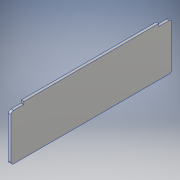
# Autodesk Inventor part: sides
Saved by Autodesk Inventor 2018.1 (Build 221171000, 171)
## iProperties
Created: 2019-02-20
Part Number: sides
Material: Aluminum 6061
Document SubType Name: Sheet Metal
Designer: RCCol
Density: 2.7 g/cm^3
Sheet Metal Rule: 3mm thick aluminum
Appearance: Aluminum - Flat
Author: RCCol
Autodesk Inventor part; units mm, degrees
ref_plane "YZ Plane" through (0, 0, 0) normal (1, 0, 0) x (0, 1, 0)
ref_plane "XZ Plane" through (0, 0, 0) normal (0, 1, 0) x (-1, 0, 0)
ref_plane "XY Plane" through (0, 0, 0) normal (0, 0, 1) x (1, 0, 0)
sketch "Sketch1" plane through (0, 0, 0) normal (1, 0, 0) x (0, 1, 0)
  line L0 (63.5, -12.7) -> (60.325, -12.7)
  line L1 (60.325, -12.7) -> (60.325, 0)
  arc A0 (60.325, 0) -> (57.15, 3.175) centre (57.15, 0) ccw
  line L2 (57.15, 3.175) -> (6.35, 3.175)
  arc A1 (6.35, 3.175) -> (3.175, 0) centre (6.35, 0) ccw
  line L3 (3.175, 0) -> (3.175, -191.77)
  arc A2 (3.175, -191.77) -> (6.35, -194.945) centre (6.35, -191.77) ccw
  line L4 (6.35, -194.945) -> (57.15, -194.945)
  arc A3 (57.15, -194.945) -> (60.325, -191.77) centre (57.15, -191.77) ccw
  line L5 (60.325, -191.77) -> (60.325, -179.07)
  line L6 (60.325, -179.07) -> (63.5, -179.07)
  line L7 (63.5, -179.07) -> (63.5, -12.7)
  line L8 (60.325, -179.07) -> (63.5, -179.07)
  line L9 (60.325, -179.07) -> (60.325, -191.77)
  line L10 (63.5, -12.7) -> (60.325, -12.7)
  line L11 (60.325, -12.7) -> (60.325, 0)
  line L12 (57.15, 3.175) -> (6.35, 3.175)
  line L13 (57.15, -194.945) -> (6.35, -194.945)
  line L14 (3.175, 0) -> (3.175, -191.77)
  arc A4 (6.35, 3.175) -> (3.175, 0) centre (6.35, 0) ccw
  arc A5 (60.325, 0) -> (57.15, 3.175) centre (57.15, 0) ccw
  point P0 (0, 0)
extrude "Plate1" add sketch "Sketch1" along normal blind 3.175
equation "\"BendRadius\" = Thickness"
equation "\"BendReliefWidth\" = Thickness"
equation "\"BendReliefDepth\" = 0.5 * Thickness"
equation "\"CornerReliefSize\" = 4 * Thickness"
equation "\"MinimumRemnant\" = 2 * Thickness"
equation "\"TransitionRadius\" = BendRadius"
equation "\"JacobiRadiusSize\" = BendRadius"
equation "\"GapSize\" = Thickness"
body "Solid1"
